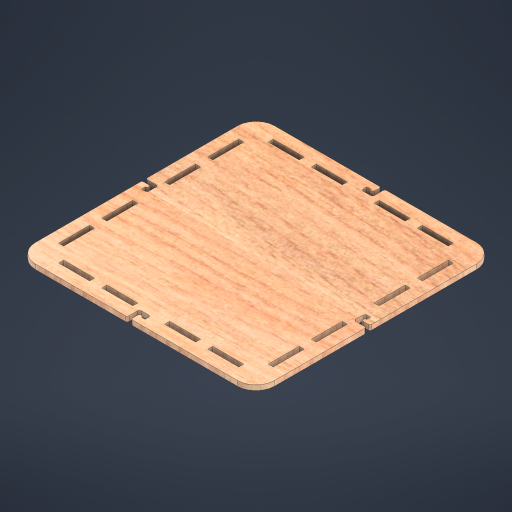
# Autodesk Inventor part: Bottom
Saved by Autodesk Inventor 2024.1 (Build 281209000, 209)
## iProperties
Created: 2024-05-23
Part Number: Bottom
Material: Wood (Birch)
Document SubType Name: Modeling
Designer: Tim Jäger
Density: 0.55 g/cm^3
Appearance: Birch - Natural Polished
Author: Tim Jäger
Autodesk Inventor part; units mm, degrees
ref_plane "YZ Plane" through (0, 0, 0) normal (1, 0, 0) x (0, 1, 0)
ref_plane "XZ Plane" through (0, 0, 0) normal (0, 1, 0) x (-1, 0, 0)
ref_plane "XY Plane" through (0, 0, 0) normal (0, 0, 1) x (1, 0, 0)
sketch "Sketch1" plane through (0, 0, 0) normal (0, 1, 0) x (-1, 0, 0)
  line L0 (-82, 97) -> (82, 97)
  line L1 (97, 82) -> (97, -82)
  line L2 (82, -97) -> (-82, -97)
  line L3 (-97, -82) -> (-97, 82)
  line L4 (-97, 97) -> (97, -97) construction
  line L5 (97, 97) -> (-97, -97) construction
  line L6 (73, -87) -> (48, -87)
  line L7 (48, -87) -> (48, -83)
  line L8 (48, -83) -> (73, -83)
  line L9 (73, -83) -> (73, -87)
  line L10 (38, -87) -> (13, -87)
  line L11 (13, -87) -> (13, -83)
  line L12 (13, -83) -> (38, -83)
  line L13 (38, -83) -> (38, -87)
  line L14 (83, -73) -> (87, -73)
  line L15 (87, -73) -> (87, -48)
  line L16 (87, -48) -> (83, -48)
  line L17 (83, -48) -> (83, -73)
  line L18 (83, -38) -> (87, -38)
  line L19 (87, -38) -> (87, -13)
  line L20 (87, -13) -> (83, -13)
  line L21 (83, -13) -> (83, -38)
  line L22 (83, 73) -> (87, 73)
  line L23 (87, 48) -> (83, 48)
  line L24 (83, 48) -> (83, 73)
  line L25 (87, 73) -> (87, 48)
  line L26 (48, 83) -> (73, 83)
  line L27 (73, 87) -> (48, 87)
  line L28 (83, 13) -> (83, 38)
  line L29 (87, 38) -> (87, 13)
  line L30 (87, 13) -> (83, 13)
  line L31 (83, 38) -> (87, 38)
  line L32 (48, 87) -> (48, 83)
  line L33 (38, 83) -> (38, 87)
  line L34 (38, 87) -> (13, 87)
  line L35 (13, 87) -> (13, 83)
  line L36 (13, 83) -> (38, 83)
  line L37 (73, 83) -> (73, 87)
  line L38 (-73, 83) -> (-73, 87)
  line L39 (-48, 87) -> (-48, 83)
  line L40 (-48, 83) -> (-73, 83)
  line L41 (-73, 87) -> (-48, 87)
  line L42 (-83, 48) -> (-83, 73)
  line L43 (-87, 73) -> (-87, 48)
  line L44 (-13, 83) -> (-38, 83)
  line L45 (-38, 87) -> (-13, 87)
  line L46 (-13, 87) -> (-13, 83)
  line L47 (-38, 83) -> (-38, 87)
  line L48 (-87, 48) -> (-83, 48)
  line L49 (-83, 38) -> (-87, 38)
  line L50 (-87, 38) -> (-87, 13)
  line L51 (-87, 13) -> (-83, 13)
  line L52 (-83, 13) -> (-83, 38)
  line L53 (-83, 73) -> (-87, 73)
  line L54 (-83, -73) -> (-87, -73)
  line L55 (-87, -48) -> (-83, -48)
  line L56 (-83, -48) -> (-83, -73)
  line L57 (-87, -73) -> (-87, -48)
  line L58 (-48, -83) -> (-73, -83)
  line L59 (-73, -87) -> (-48, -87)
  line L60 (-83, -13) -> (-83, -38)
  line L61 (-87, -38) -> (-87, -13)
  line L62 (-87, -13) -> (-83, -13)
  line L63 (-83, -38) -> (-87, -38)
  line L64 (-48, -87) -> (-48, -83)
  line L65 (-38, -83) -> (-38, -87)
  line L66 (-38, -87) -> (-13, -87)
  line L67 (-13, -87) -> (-13, -83)
  line L68 (-13, -83) -> (-38, -83)
  line L69 (-73, -83) -> (-73, -87)
  arc A0 (82, -97) -> (97, -82) centre (82, -82) ccw
  arc A1 (-97, -82) -> (-82, -97) centre (-82, -82) ccw
  arc A2 (-82, 97) -> (-97, 82) centre (-82, 82) ccw
  arc A3 (97, 82) -> (82, 97) centre (82, 82) ccw
  line L70 (97, -7.5) -> (87, -7.5)
  line L71 (87, -7.5) -> (87, 1.5)
  line L72 (87, 1.5) -> (90, 1.5)
  line L73 (90, 1.5) -> (90, -1.5) construction
  line L74 (90, -4.5) -> (97, -4.5)
  line L75 (90, 1.5) -> (91.5, 1.5)
  line L76 (91.5, 1.5) -> (91.5, -1.5)
  line L77 (91.5, -1.5) -> (90, -1.5)
  line L78 (90, -1.5) -> (90, 1.5) construction
  line L79 (90, -1.5) -> (90, -4.5)
  line L80 (-1.5, 87) -> (-1.5, 90)
  line L81 (-1.5, 90) -> (-1.5, 91.5)
  line L82 (-1.5, 90) -> (1.5, 90) construction
  line L83 (1.5, 90) -> (-1.5, 90) construction
  line L84 (-1.5, 91.5) -> (1.5, 91.5)
  line L85 (1.5, 90) -> (4.5, 90)
  line L86 (7.5, 87) -> (-1.5, 87)
  line L87 (4.5, 90) -> (4.5, 97)
  line L88 (7.5, 97) -> (7.5, 87)
  line L89 (1.5, 91.5) -> (1.5, 90)
  line L90 (-87, -1.5) -> (-90, -1.5)
  line L91 (-90, -1.5) -> (-91.5, -1.5)
  line L92 (-90, -1.5) -> (-90, 1.5) construction
  line L93 (-90, 1.5) -> (-90, -1.5) construction
  line L94 (-91.5, -1.5) -> (-91.5, 1.5)
  line L95 (-90, 1.5) -> (-90, 4.5)
  line L96 (-87, 7.5) -> (-87, -1.5)
  line L97 (-90, 4.5) -> (-97, 4.5)
  line L98 (-97, 7.5) -> (-87, 7.5)
  line L99 (-91.5, 1.5) -> (-90, 1.5)
  line L100 (1.5, -87) -> (1.5, -90)
  line L101 (1.5, -90) -> (1.5, -91.5)
  line L102 (1.5, -90) -> (-1.5, -90) construction
  line L103 (-1.5, -90) -> (1.5, -90) construction
  line L104 (1.5, -91.5) -> (-1.5, -91.5)
  line L105 (-1.5, -90) -> (-4.5, -90)
  line L106 (-7.5, -87) -> (1.5, -87)
  line L107 (-4.5, -90) -> (-4.5, -97)
  line L108 (-7.5, -97) -> (-7.5, -87)
  line L109 (-1.5, -91.5) -> (-1.5, -90)
  point P0 (0, 0)
  point P1 (73, -85)
  point P2 (85, -38)
  point P3 (85, -48)
  point P4 (85, -13)
  point P5 (85, 73)
  point P6 (48, 85)
  point P7 (38, 85)
  point P8 (13, 85)
  point P9 (-73, 85)
  point P10 (-85, 48)
  point P11 (-85, 38)
  point P12 (-85, 13)
  point P13 (-85, -73)
  point P14 (-48, -85)
  point P15 (-38, -85)
  point P16 (-13, -85)
  point P17 (92, -7.5)
  point P18 (91.5, 0)
  point P19 (0, 91.5)
  point P20 (7.5, 92)
  point P21 (-91.5, 0)
  point P22 (-92, 7.5)
  point P23 (0, -91.5)
  point P24 (-7.5, -92)
  point P25 (7.5, 97)
  point P26 (4.5, 97)
  point P27 (-97, 7.5)
  point P28 (-97, 4.5)
  point P29 (-7.5, -97)
  point P30 (-4.5, -97)
  dimension "d0" = 25
  dimension "d1" = 4
  dimension "d4" = 10
  dimension "d5" = 13
  dimension "d6" = 10
  dimension "d7" = 10
  dimension "d8" = 10
  dimension "d9" = 13
  dimension "d12" = 360
  dimension "d14" = 10
  dimension "d15" = 10
  dimension "d16" = 15
  dimension "d17" = 7
  dimension "d18" = 3
  dimension "d19" = 6
  dimension "d20" = 3
  dimension "d21" = 1.5
  dimension "d24" = 360
  constraints: 220 end point, 14 point on line, 12 parallel, 11 perpendicular, 8 midpoint, 8 point on circle, 8 tangent, 7 horizontal, 6 equal length, 4 centre point, 3 equal radius, 2 vertical alignment, 1 horizontal alignment, 230 other
  measures "d0" distance of L7.end L8.end
  measures "d1" distance of L6.end L7.end
  measures "d4" distance of L6.end L10.start
  measures "d5" horizontal distance of point (0, 0) L10.end
  measures "d6" distance from line of L14.start L8
  measures "d7" distance from line of point (73, -85) L17
  measures "d8" distance of point (85, -38) point (85, -48)
  measures "d9" vertical distance of point (0, 0) point (85, -13)
  measures "d14" distance between parallel lines of L2 L10
  measures "d15" distance between parallel lines of L3 L57
  measures "d16" radius of A0
  measures "d17" distance between parallel lines of L1 L73
  measures "d18" distance from line of point (92, -7.5) L74
  measures "d19" distance of L72.end L74.start
  measures "d20" distance of L75.end L76.end
  measures "d21" distance of L76.end L73.end
extrude "Extrusion1" add sketch "Sketch1" along normal blind 4 contours L0 L87 L85 L89 L84 L81 L80 L86 L88 A3 L1 L74 L79 L77 L76 L75 L72 L71 L70 A0 L2 L107 L105 L109 L104 L101 L100 L106 L108 A1 L3 L97 L95 L99 L94 L91 L90 L96 L98 A2
fillet "Fillet1" radius 1.5 24 edges at (-4.5, 2, 97) (-7.5, 2, 97) (-7.5, 2, 87) (-4.5, 2, 90) (1.5, 2, 87) (-1.5, 2, 90) (87, 2, 7.5) (97, 2, 7.5) (97, 2, 4.5) (90, 2, 4.5) (90, 2, 1.5) (87, 2, -1.5) (-1.5, 2, -87) (1.5, 2, -90) (4.5, 2, -90) (7.5, 2, -87) (4.5, 2, -97) (7.5, 2, -97) (-97, 2, -4.5) (-97, 2, -7.5) (-90, 2, -4.5) (-90, 2, -1.5) (-87, 2, 1.5) (-87, 2, -7.5)
equation "\"d6\" = d7"
equation "\"d8\" = d4"
equation "\"d15\" = d14"
body "Solid1"
